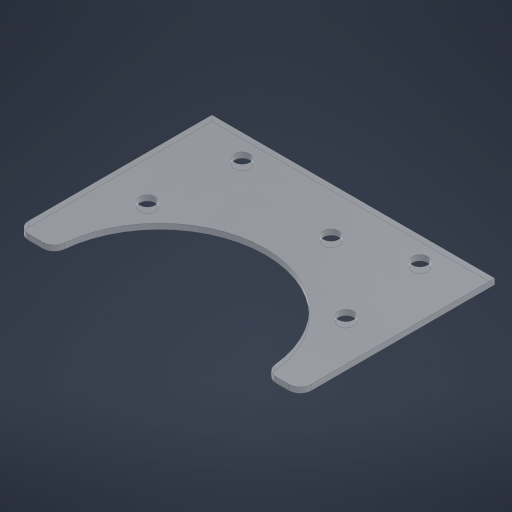
# Autodesk Inventor part: Winter-Climb-Guides
Saved by Autodesk Inventor 2024 (Build 280153000, 153)
## iProperties
Created: 2024-01-17
Part Number: Winter-Climb-Guides
Material: Polycarbonate, Clear
Document SubType Name: Sheet Metal
Designer: abhin
Density: 1.2 g/cm^3
Appearance: Polycarbonate - Clear
Flat Pattern Width: 5.5626 cm
Flat Pattern Length: 8.08228 cm
Flat Pattern Area: 44.9585 cm^2
Sheet Metal Rule: Default
Sheet Metal Width: 2.190 in
Sheet Metal Length: 3.182 in
Sheet Metal Area: 6.969 in^2
Author: abhin
Autodesk Inventor part; units mm, degrees
ref_plane "YZ Plane" through (0, 0, 0) normal (1, 0, 0) x (0, 1, 0)
ref_plane "XZ Plane" through (0, 0, 0) normal (0, 1, 0) x (-1, 0, 0)
ref_plane "XY Plane" through (0, 0, 0) normal (0, 0, 1) x (1, 0, 0)
sketch "Sketch1" plane through (0, 0, 0) normal (0, 1, 0) x (-1, 0, 0)
  line L0 (46.76465, 19.785927) -> (46.76465, -5.614073)
  line L1 (46.76465, -5.614073) -> (-34.05815, -5.614073)
  line L2 (-34.05815, -5.614073) -> (-34.05815, 19.785927)
  line L3 (-34.05815, 19.785927) -> (46.76465, -5.614073) construction
  line L4 (46.76465, 19.785927) -> (-34.05815, -5.614073) construction
  line L5 (-34.05815, 19.785927) -> (-34.05815, 50.011927)
  line L6 (46.76465, 19.785927) -> (46.76465, 50.011927)
  line L7 (46.76465, 19.785927) -> (-34.05815, 19.785927)
  line L8 (46.76465, 19.785927) -> (6.35325, 19.785927)
  line L9 (46.76465, 50.011927) -> (37.59525, 50.011927)
  line L10 (-23.87275, 50.011927) -> (-34.05815, 50.011927)
  line L11 (37.59525, 50.011927) -> (36.32525, 50.011927)
  arc A0 (-24.12675, 50.011927) -> (36.32525, 50.011927) centre (6.09925, 50.011927) ccw
  point P0 (6.35325, 7.085927)
  dimension "d11" = 80.8228
  dimension "d12" = 25.4
  dimension "d13" = 30.226
  dimension "d14" = 30.226
  dimension "d40" = 40.4114
  dimension "d46" = 60.452
  constraints: 24 end point, 3 midpoint, 2 horizontal, 2 point on circle, 2 vertical, 1 centre point, 1 collinear, 1 parallel, 1 point on line
  measures "d11" distance of L0.end L1.end
  measures "d12" distance of L1.end L2.end
  measures "d13" distance of L2.end L5.end
  measures "d14" distance of L0.start L6.end
  measures "d40" distance of L0.start L8.end
  measures "d46" diameter of A0
sketch "Sketch1 outline for Extrusion3" plane through (0, 0, 0) normal (0, 1, 0) x (-1, 0, 0)
  line L0 (-34.05815, 50.011927) -> (-34.05815, 19.785927)
  line L1 (-24.12675, 50.011927) -> (-34.05815, 50.011927)
  arc A0 (36.32525, 50.011927) -> (-24.12675, 50.011927) centre (6.09925, 50.011927) cw
  line L2 (37.59525, 50.011927) -> (36.32525, 50.011927)
  line L3 (46.76465, 50.011927) -> (37.59525, 50.011927)
  line L4 (46.76465, 19.785927) -> (46.76465, 50.011927)
  line L5 (46.76465, -5.614073) -> (46.76465, 19.785927)
  line L6 (-34.05815, -5.614073) -> (46.76465, -5.614073)
  line L7 (-34.05815, 19.785927) -> (-34.05815, -5.614073)
extrude "Extrusion3" add sketch "Sketch1 outline for Extrusion3" along normal blind 1.5875
sketch "Sketch2" plane through (0, 1.5875, 0) normal (0, 1, 0) x (1, 0, 0)
  line L0 (34.05815, 5.614073) -> (-46.76465, 5.614073)
  line L1 (34.05815, 5.614073) -> (34.05815, -19.785927)
  line L2 (34.05815, -50.011927) -> (34.05815, 5.614073)
  line L3 (34.05815, 5.614073) -> (34.05815, -0.735927)
  line L4 (34.05815, -0.735927) -> (19.04675, -0.735927)
  circle A0 centre (19.04675, -0.735927) radius 2.1844
  line L5 (34.05815, 5.614073) -> (34.05815, -7.085927)
  line L6 (34.05815, -7.085927) -> (-0.00325, -7.085927)
  circle A1 centre (-0.00325, -7.085927) radius 2.1844
  line L7 (19.04675, -0.735927) -> (-31.75325, -0.735927)
  circle A2 centre (-31.75325, -0.735927) radius 2.1844
  arc A3 (-46.76465, -56.057127) -> (-44.93585, -57.885927) centre (-44.93585, -56.057127) ccw
  arc A4 (32.22935, -57.885927) -> (34.05815, -56.057127) centre (32.22935, -56.057127) ccw
  line L8 (34.05815, -19.785927) -> (-46.76465, -19.785927)
  line L9 (-46.76465, 5.614073) -> (-46.76465, -50.011927)
  line L10 (34.05815, -19.785927) -> (34.05815, -24.865927)
  line L11 (34.05815, -24.865927) -> (21.99315, -24.865927)
  circle A5 centre (21.99315, -24.865927) radius 2.1844
  line L12 (-46.76465, -19.785927) -> (-46.76465, -24.865927)
  line L13 (-46.76465, -24.865927) -> (-34.69965, -24.865927)
  circle A6 centre (-34.69965, -24.865927) radius 2.1844
  point P0 (0, 0)
  point P1 (-31.057127, -40.306856)
  point P2 (31.050628, -40.30613)
  point P3 (-43.267434, -44.121852)
  point P4 (30.560934, -44.122114)
  dimension "d18" = 25.4
  dimension "d19" = 6.35
  dimension "d20" = 15.0114
  dimension "d21" = 4.3688
  dimension "d22" = 12.7
  dimension "d23" = 34.0614
  dimension "d24" = 4.3688
  dimension "d25" = 50.8
  dimension "d26" = 4.3688
  dimension "d30" = 5.08
  dimension "d31" = 12.065
  dimension "d32" = 4.3688
  dimension "d33" = 5.08
  dimension "d34" = 12.065
  dimension "d35" = 4.3688
  constraints: 22 end point, 6 point on line, 5 centre point, 5 coincident, 3 horizontal, 3 perpendicular
  measures "d18" distance of L0.start L1.end
  measures "d19" distance of L0.start L3.end
  measures "d20" distance of L3.end L4.end
  measures "d21" diameter of A0
  measures "d22" distance of L0.start L5.end
  measures "d23" distance of L5.end L6.end
  measures "d24" diameter of A1
  measures "d25" distance of L7.start L7.end
  measures "d26" diameter of A2
  measures "d30" distance of L1.end L10.end
  measures "d31" distance of L10.end L11.end
  measures "d32" diameter of A5
  measures "d33" distance of L8.end L12.end
  measures "d34" distance of L12.end L13.end
  measures "d35" diameter of A6
extrude "Extrusion4" cut sketch "Sketch2" against normal blind 1.5875 contours A0 L7 L4 | L4 L7 A0 | A1 | A2 | A5 | A6
fillet "Fillet2" radius 3.175 4 edges at (-46.7646, 0.7937, 50.0119) (34.0582, 0.7937, 50.0119) (-36.3252, 0.7937, 50.0119) (24.1268, 0.7937, 50.0119)
equation "\"d31\" = d34"
equation "\"BendRadius\" = Thickness"
equation "\"BendReliefWidth\" = Thickness"
equation "\"BendReliefDepth\" = 0.5 * Thickness"
equation "\"CornerReliefSize\" = 4 * Thickness"
equation "\"MinimumRemnant\" = 2 * Thickness"
equation "\"TransitionRadius\" = BendRadius"
equation "\"JacobiRadiusSize\" = BendRadius"
equation "\"GapSize\" = Thickness"
equation "\"Thickness\" = 1.5875"
body "Solid3"
